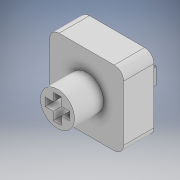
# Autodesk Inventor part: IPC M-SEL 0 key
Saved by Autodesk Inventor 2022 (Build 260153000, 153)
## iProperties
Created: 2021-12-31
Part Number: IPC M-SEL 0 key
Material: Generic
Document SubType Name: Modeling
Designer: solor
Density: 1 g/cm^3
Appearance: Default
Author: solor
Autodesk Inventor part; units mm, degrees
ref_plane "YZ Plane" through (0, 0, 0) normal (1, 0, 0) x (0, 1, 0)
ref_plane "XZ Plane" through (0, 0, 0) normal (0, 1, 0) x (-1, 0, 0)
sketch "Sketch1" plane through (0, 0, 0) normal (0, 0, 1) x (1, 0, 0)
  line L0 (14.6962, 12.74) -> (14.6962, 0) construction
  line L1 (10.61, 12.2) -> (1.53, 12.2)
  arc A0 (1.53, 12.2) -> (0, 10.67) centre (1.53, 10.67) ccw
  line L2 (0, 10.67) -> (0, 1.53)
  arc A1 (0, 1.53) -> (1.53, 0) centre (1.53, 1.53) ccw
  line L3 (1.53, 0) -> (10.61, 0)
  arc A2 (10.61, 0) -> (12.14, 1.53) centre (10.61, 1.53) ccw
  arc A3 (12.14, 10.67) -> (10.61, 12.2) centre (10.61, 10.67) ccw
  line L4 (12.14, 10.67) -> (12.14, 1.53)
  point P0 (0, 0)
  point P1 (0, 0)
  dimension "d10" = 12.74
  constraints: 10 end point, 8 point on circle, 4 centre point, 2 vertical, 1 point on line
  measures "d10" distance of L0.start L0.end
ref_plane "Work Plane1" through (0, 0, 5) normal (0, 0, 1) x (1, 0, 0)
sketch "Sketch2" plane through (0, 0, 5) normal (0, 0, 1) x (1, 0, 0)
  line L0 (10.88, 12.74) -> (1.8, 12.74) projected
  line L1 (10.88, 12.74) -> (1.8, 12.74) projected
  arc A0 (1.8, 12.74) -> (0, 10.94) centre (1.8, 10.94) ccw projected
  line L2 (0, 10.94) -> (0, 1.8) projected
  arc A1 (0, 1.8) -> (1.8, 0) centre (1.8, 1.8) ccw projected
  line L3 (1.8, 0) -> (10.88, 0) projected
  arc A2 (10.88, 0) -> (12.68, 1.8) centre (10.88, 1.8) ccw projected
  line L4 (12.68, 1.8) -> (12.68, 10.94) projected
  arc A3 (12.68, 10.94) -> (10.88, 12.74) centre (10.88, 10.94) ccw projected
  circle A4 centre (6.34, 6.37) radius 2.8
  line L5 (5.665, 8.395) -> (7.015, 8.395)
  line L6 (7.015, 4.345) -> (5.665, 4.345)
  line L7 (5.665, 4.345) -> (7.015, 8.395) construction
  line L8 (5.665, 8.395) -> (7.015, 4.345) construction
  line L9 (8.365, 5.695) -> (8.365, 7.045)
  line L10 (4.315, 7.045) -> (4.315, 5.695)
  line L11 (4.315, 5.695) -> (8.365, 7.045) construction
  line L12 (8.365, 5.695) -> (4.315, 7.045) construction
  line L13 (4.315, 5.695) -> (5.665, 5.695)
  line L14 (7.015, 5.695) -> (8.365, 5.695)
  line L15 (5.665, 4.345) -> (5.665, 5.695)
  line L16 (5.665, 7.045) -> (5.665, 8.395)
  line L17 (8.365, 7.045) -> (7.015, 7.045)
  line L18 (5.665, 7.045) -> (4.315, 7.045)
  line L19 (7.015, 8.395) -> (7.015, 7.045)
  line L20 (7.015, 5.695) -> (7.015, 4.345)
  point P0 (0, 0)
  dimension "d3" = 5.6
  dimension "d4" = 4.05
  dimension "d5" = 1.35
  dimension "d6" = 4.05
  dimension "d7" = 1.35
  constraints: 32 end point, 10 parallel, 8 perpendicular, 4 midpoint, 2 vertical, 1 centre point
  measures "d3" diameter of A4
  measures "d4" distance of L6.end L5.start
  measures "d5" distance of L5.start L5.end
  measures "d6" distance of L10.end L9.start
  measures "d7" distance of L9.end L9.start
extrude "Extrusion3" add sketch "Sketch1" along normal blind 5
sketch "Sketch3" plane through (0, 0, 5) normal (0, 0, 1) x (1, 0, 0)
  line L0 (10.61, 12.47) -> (1.53, 12.47)
  line L1 (10.61, 12.47) -> (1.53, 12.47)
  arc A0 (1.53, 12.47) -> (-0.27, 10.67) centre (1.53, 10.67) ccw
  line L2 (-0.27, 10.67) -> (-0.27, 1.53)
  arc A1 (-0.27, 1.53) -> (1.53, -0.27) centre (1.53, 1.53) ccw
  line L3 (1.53, -0.27) -> (10.61, -0.27)
  arc A2 (10.61, -0.27) -> (12.41, 1.53) centre (10.61, 1.53) ccw
  line L4 (12.41, 1.53) -> (12.41, 10.67)
  arc A3 (12.41, 10.67) -> (10.61, 12.47) centre (10.61, 10.67) ccw
  circle A4 centre (6.07, 6.1) radius 2.8
  line L5 (5.395, 8.125) -> (6.745, 8.125)
  line L6 (6.745, 4.075) -> (5.395, 4.075)
  line L7 (5.395, 4.075) -> (6.745, 8.125) construction
  line L8 (5.395, 8.125) -> (6.745, 4.075) construction
  line L9 (8.095, 5.425) -> (8.095, 6.775)
  line L10 (4.045, 6.775) -> (4.045, 5.425)
  line L11 (4.045, 5.425) -> (8.095, 6.775) construction
  line L12 (8.095, 5.425) -> (4.045, 6.775) construction
  line L13 (4.045, 5.425) -> (5.395, 5.425)
  line L14 (6.745, 5.425) -> (8.095, 5.425)
  line L15 (5.395, 4.075) -> (5.395, 5.425)
  line L16 (5.395, 6.775) -> (5.395, 8.125)
  line L17 (8.095, 6.775) -> (6.745, 6.775)
  line L18 (5.395, 6.775) -> (4.045, 6.775)
  line L19 (6.745, 8.125) -> (6.745, 6.775)
  line L20 (6.745, 5.425) -> (6.745, 4.075)
  line L21 (10.61, 12.2) -> (1.53, 12.2) projected
  line L22 (0, 10.67) -> (0, 1.53) projected
  point P0 (0, 0)
  point P1 (-0.27, -0.27)
  point P2 (6.07, 12.2)
  point P3 (0, 6.1)
  point P4 (6.07, 6.1)
  dimension "d14" = 5.6
  dimension "d15" = 4.05
  dimension "d16" = 1.35
  dimension "d17" = 4.05
  dimension "d18" = 1.35
  constraints: 42 end point, 10 parallel, 8 perpendicular, 8 point on circle, 6 midpoint, 5 centre point, 2 vertical
  measures "d14" diameter of A4
  measures "d15" distance of L6.end L5.start
  measures "d16" distance of L5.start L5.end
  measures "d17" distance of L10.end L9.start
  measures "d18" distance of L9.end L9.start
extrude "Extrusion4" add sketch "Sketch3" along normal blind 4.8 contours A4
sketch "Sketch4" plane through (0, 0, 0) normal (0, 0, -1) x (-1, 0, 0)
  line L0 (-13.9436, 0) -> (-13.9436, 2.266)
  line L1 (-15.5559, 0) -> (-15.5559, 6.84)
  line L2 (-1.53, 0) -> (-10.61, 0) projected
  line L3 (-11.9098, 9.6363) -> (-0.2302, 9.6363) construction
  line L4 (-0.2302, 9.6363) -> (-0.2302, 6.84) construction
  line L5 (-0.2302, 6.84) -> (-11.9098, 6.84) construction
  line L6 (-11.9098, 6.84) -> (-11.9098, 9.6363) construction
  line L7 (-7.4059, 5.4421) -> (-4.7341, 5.4421) construction
  line L8 (-4.7341, 5.4421) -> (-4.7341, 2.266) construction
  line L9 (-4.7341, 2.266) -> (-7.4059, 2.266) construction
  line L10 (-7.4059, 2.266) -> (-7.4059, 5.4421) construction
  line L11 (-8.8728, 6.8881) -> (-9.5467, 6.8881)
  line L12 (-9.5467, 6.8881) -> (-9.5467, 8.6779)
  line L13 (-9.5467, 8.6779) -> (-10.0369, 7.5227)
  line L14 (-10.0369, 7.5227) -> (-10.5007, 7.5227)
  line L15 (-10.5007, 7.5227) -> (-10.9908, 8.6779)
  line L16 (-10.9908, 8.6779) -> (-10.9908, 6.8881)
  line L17 (-10.9908, 6.8881) -> (-11.6297, 6.8881)
  line L18 (-11.6297, 6.8881) -> (-11.6297, 9.5881)
  line L19 (-11.6297, 9.5881) -> (-10.8486, 9.5881)
  line L20 (-10.8486, 9.5881) -> (-10.2491, 8.2556)
  line L21 (-10.2491, 8.2556) -> (-9.654, 9.5881)
  line L22 (-9.654, 9.5881) -> (-8.8728, 9.5881)
  line L23 (-8.8728, 9.5881) -> (-8.8728, 6.8881)
  line L24 (-7.1924, 7.829) -> (-8.3937, 7.829)
  line L25 (-8.3937, 7.829) -> (-8.3937, 8.3322)
  line L26 (-8.3937, 8.3322) -> (-7.1924, 8.3322)
  line L27 (-7.1924, 8.3322) -> (-7.1924, 7.829)
  spline S0 degree 2 poles (-5.8775, 6.84) (-6.1882, 6.84) (-6.6564, 6.9603) (-6.8577, 7.0479) knots 0 0 0 1 2 2 2
  line L28 (-6.8577, 7.0479) -> (-6.8577, 7.6911)
  line L29 (-6.8577, 7.6911) -> (-6.7964, 7.6911)
  spline S1 degree 2 poles (-6.7964, 7.6911) (-6.5929, 7.5183) (-6.105, 7.3323) (-5.8753, 7.3323) knots 0 0 0 1 2 2 2
  spline S2 degree 2 poles (-5.8753, 7.3323) (-5.8162, 7.3323) (-5.6258, 7.3586) (-5.5689, 7.3848) knots 0 0 0 1 2 2 2
  spline S3 degree 2 poles (-5.5689, 7.3848) (-5.4989, 7.4154) (-5.4005, 7.527) (-5.4005, 7.6167) knots 0 0 0 1 2 2 2
  spline S4 degree 2 poles (-5.4005, 7.6167) (-5.4005, 7.7196) (-5.5602, 7.8465) (-5.6696, 7.8749) knots 0 0 0 1 2 2 2
  spline S5 degree 2 poles (-5.6696, 7.8749) (-5.8074, 7.9121) (-6.1203, 7.9756) (-6.2582, 8.0237) knots 0 0 0 1 2 2 2
  spline S6 degree 2 poles (-6.2582, 8.0237) (-6.5711, 8.1331) (-6.8424, 8.5073) (-6.8424, 8.7873) knots 0 0 0 1 2 2 2
  spline S7 degree 2 poles (-6.8424, 8.7873) (-6.8424, 9.1659) (-6.2013, 9.6363) (-5.7199, 9.6363) knots 0 0 0 1 2 2 2
  spline S8 degree 2 poles (-5.7199, 9.6363) (-5.4792, 9.6363) (-5.0023, 9.5378) (-4.8141, 9.4547) knots 0 0 0 1 2 2 2
  line L30 (-4.8141, 9.4547) -> (-4.8141, 8.8377)
  line L31 (-4.8141, 8.8377) -> (-4.8732, 8.8377)
  spline S9 degree 2 poles (-4.8732, 8.8377) (-5.0241, 8.9667) (-5.4574, 9.144) (-5.6849, 9.144) knots 0 0 0 1 2 2 2
  spline S10 degree 2 poles (-5.6849, 9.144) (-5.7746, 9.144) (-5.9147, 9.1177) (-5.9934, 9.0827) knots 0 0 0 1 2 2 2
  spline S11 degree 2 poles (-5.9934, 9.0827) (-6.0569, 9.0543) (-6.1488, 8.9405) (-6.1488, 8.8705) knots 0 0 0 1 2 2 2
  spline S12 degree 2 poles (-6.1488, 8.8705) (-6.1488, 8.7654) (-6.0022, 8.6451) (-5.7921, 8.597) knots 0 0 0 1 2 2 2
  spline S13 degree 2 poles (-5.7921, 8.597) (-5.6565, 8.5663) (-5.4048, 8.5073) (-5.2604, 8.4569) knots 0 0 0 1 2 2 2
  spline S14 degree 2 poles (-5.2604, 8.4569) (-4.9804, 8.3541) (-4.7069, 8.0128) (-4.7069, 7.7327) knots 0 0 0 1 2 2 2
  spline S15 degree 2 poles (-4.7069, 7.7327) (-4.7069, 7.3301) (-5.3392, 6.84) (-5.8775, 6.84) knots 0 0 0 1 2 2 2
  line L32 (-4.359, 6.8881) -> (-4.359, 9.5881)
  line L33 (-4.359, 9.5881) -> (-2.5342, 9.5881)
  line L34 (-2.5342, 9.5881) -> (-2.5342, 9.074)
  line L35 (-2.5342, 9.074) -> (-3.6851, 9.074)
  line L36 (-3.6851, 9.074) -> (-3.6851, 8.5992)
  line L37 (-3.6851, 8.5992) -> (-2.6239, 8.5992)
  line L38 (-2.6239, 8.5992) -> (-2.6239, 8.085)
  line L39 (-2.6239, 8.085) -> (-3.6851, 8.085)
  line L40 (-3.6851, 8.085) -> (-3.6851, 7.4023)
  line L41 (-3.6851, 7.4023) -> (-2.5342, 7.4023)
  line L42 (-2.5342, 7.4023) -> (-2.5342, 6.8881)
  line L43 (-2.5342, 6.8881) -> (-4.359, 6.8881)
  line L44 (-0.274, 6.8881) -> (-2.0747, 6.8881)
  line L45 (-2.0747, 6.8881) -> (-2.0747, 9.5881)
  line L46 (-2.0747, 9.5881) -> (-1.3964, 9.5881)
  line L47 (-1.3964, 9.5881) -> (-1.3964, 7.4023)
  line L48 (-1.3964, 7.4023) -> (-0.274, 7.4023)
  line L49 (-0.274, 7.4023) -> (-0.274, 6.8881)
  spline S16 degree 2 poles (-4.8947, 3.8553) (-4.8947, 3.4598) (-5.0208, 2.8666) (-5.1617, 2.6664) knots 0 0 0 1 2 2 2
  spline S17 degree 2 poles (-5.1617, 2.6664) (-5.3001, 2.4687) (-5.7475, 2.266) (-6.0688, 2.266) knots 0 0 0 1 2 2 2
  spline S18 degree 2 poles (-6.0688, 2.266) (-6.3925, 2.266) (-6.8374, 2.4687) (-6.9783, 2.6713) knots 0 0 0 1 2 2 2
  spline S19 degree 2 poles (-6.9783, 2.6713) (-7.1192, 2.8716) (-7.2453, 3.4598) (-7.2453, 3.8553) knots 0 0 0 1 2 2 2
  spline S20 degree 2 poles (-7.2453, 3.8553) (-7.2453, 4.2606) (-7.1192, 4.834) (-6.9759, 5.0416) knots 0 0 0 1 2 2 2
  spline S21 degree 2 poles (-6.9759, 5.0416) (-6.8325, 5.2443) (-6.3802, 5.4421) (-6.0688, 5.4421) knots 0 0 0 1 2 2 2
  spline S22 degree 2 poles (-6.0688, 5.4421) (-5.74, 5.4421) (-5.3001, 5.2344) (-5.1592, 5.0293) knots 0 0 0 1 2 2 2
  spline S23 degree 2 poles (-5.1592, 5.0293) (-5.0208, 4.8291) (-4.8947, 4.2384) (-4.8947, 3.8553) knots 0 0 0 1 2 2 2
  spline S24 degree 2 poles (-5.6634, 3.8553) (-5.6634, 4.4213) (-5.8488, 4.8785) (-6.0688, 4.8785) knots 0 0 0 1 2 2 2
  spline S25 degree 2 poles (-6.0688, 4.8785) (-6.2887, 4.8785) (-6.4766, 4.4213) (-6.4766, 3.8528) knots 0 0 0 1 2 2 2
  spline S26 degree 2 poles (-6.4766, 3.8528) (-6.4766, 3.2942) (-6.2887, 2.8295) (-6.0688, 2.8295) knots 0 0 0 1 2 2 2
  spline S27 degree 2 poles (-6.0688, 2.8295) (-5.8513, 2.8295) (-5.6634, 3.2942) (-5.6634, 3.8553) knots 0 0 0 1 2 2 2
  point P0 (0, 0)
  point P1 (-6.07, 0)
  point P2 (-6.07, 2.266)
  point P3 (-6.07, 6.84)
  point P4 (-6.07, 6.84)
  point P5 (-6.07, 2.266)
  dimension "d21" = 2.266
  dimension "d22" = 6.84
  constraints: 4 end point, 3 midpoint, 2 vertical, 4 other
  measures "d21" distance of L0.start L0.end
  measures "d22" distance of L1.start L1.end
extrude "Extrusion5" add sketch "Sketch4" along normal blind 0.9
body "Solid2"
